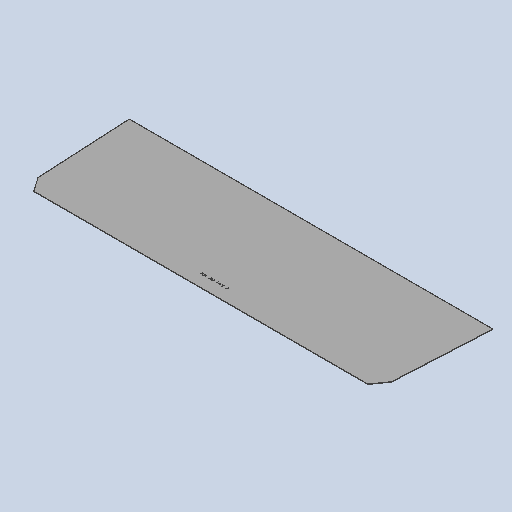
# Autodesk Inventor part: MSC 703 FACE 3
Saved by Autodesk Inventor 2025 (Build 290162010, 162A)
## iProperties
Created: 2024-06-16
Part Number: MSC 703 FACE 3
Material: AISI304
Document SubType Name: Sheet Metal
Designer: admin
Density: 8 g/cm^3
Sheet Metal Rule: AISI304 2mm Die16
Appearance: Default
Stock Number: МОО 703 морда 2
Flat Pattern Width: 163.344 cm
Flat Pattern Length: 89.2448 cm
Flat Pattern Area: 14577.6 cm^2
Sheet Metal Width: 1633,437 mm
Sheet Metal Length: 892,448 mm
Sheet Metal Area: 1457757,595 mm^2
Mass: 12180.1 g
Surface Area: 15306.4 cm^2
Volume: 1522.51 cm^3
Author: admin
Autodesk Inventor part; units mm, degrees
ref_plane "YZ Plane" through (0, 0, 0) normal (1, 0, 0) x (0, 1, 0)
ref_plane "XZ Plane" through (0, 0, 0) normal (0, 1, 0) x (-1, 0, 0)
ref_plane "XY Plane" through (0, 0, 0) normal (0, 0, 1) x (1, 0, 0)
sketch "Sketch1" plane through (0, 0, 0) normal (0, 0, 1) x (1, 0, 0)
  line L0 (800, 0) -> (800, -485) construction
  line L1 (800, -485) -> (0, -485)
  line L2 (800, 0) -> (777.7845, -423.8974)
  line L3 (735, -485) -> (800, -392.1704)
  line L4 (0, -485) -> (0, 0)
  line L5 (0, 0) -> (800, 0)
  dimension "d9" = 800
  dimension "d10" = 35
  dimension "d11" = 485
  dimension "d12" = 3
  dimension "d13" = 65
  measures "d9" distance of L4.end L0.start
  measures "d10" angle of L0 L3
  measures "d11" distance between parallel lines of L5 L1
  measures "d12" angle of L0 L2
  measures "d13" distance of L0.end L3.start
extrude "Plate1" add sketch "Sketch1" along normal blind 2
mirror "Mirror1" about plane through (0, 0, 0) normal (1, 0, 0)
sketch "Sketch2" plane through (0, 0, 2) normal (0, 0, 1) x (1, 0, 0)
  line L0 (-55, -435) -> (-55, -423) construction
  line L1 (-55, -423) -> (55, -423) construction
  line L2 (55, -423) -> (55, -435) construction
  line L3 (55, -435) -> (-55, -435) construction
  line L4 (-735, -485) -> (735, -485) projected
  point P0 (0, 0)
  point P1 (0, -435)
  point P2 (0, -485)
  dimension "d6" = 12
  dimension "d7" = 110
  dimension "d8" = 50
  constraints: 2 midpoint, 1 parallel, 1 vertical alignment, 2 other
  measures "d6" distance of L1.end L2.end
  measures "d7" distance between parallel lines of L0 L2
  measures "d8" distance between parallel lines of L4 L3
mark "Mark1"
equation "\"d2\" = Thickness"
equation "\"BendReliefWidth\" = Thickness"
equation "\"BendReliefDepth\" = 0.5 * Thickness"
equation "\"CornerReliefSize\" = 4 * Thickness"
equation "\"MinimumRemnant\" = 2 * Thickness"
equation "\"TransitionRadius\" = BendRadius"
equation "\"JacobiRadiusSize\" = BendRadius"
equation "\"GapSize\" = Thickness"
equation "\"Thickness\" = 2"
equation "\"BendRadius\" = 2.75"
body "Solid1"
